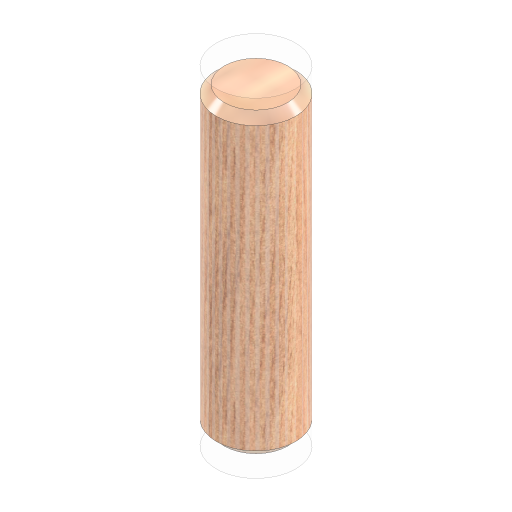
# Autodesk Inventor part: MS Dowel
Saved by Autodesk Inventor 2023 (Build 270158000, 158)
## iProperties
Created: 2024-03-28
Part Number: MS Dowel
Material: Wood (Birch)
Document SubType Name: Modeling
Designer: SauliusD
Density: 0.55 g/cm^3
Appearance: Birch - Natural Polished
Author: SauliusD
Autodesk Inventor part; units mm, degrees
ref_plane "YZ Plane" through (0, 0, 0) normal (1, 0, 0) x (0, 1, 0)
ref_plane "XZ Plane" through (0, 0, 0) normal (0, 1, 0) x (-1, 0, 0)
sketch "Sketch1" plane through (0, 0, 0) normal (0, 0, 1) x (1, 0, 0)
  circle A0 centre (0, 0) radius 4
  dimension "Diam" = 8
  constraints: 1 centre point, 1 coincident
  measures "Diam" diameter of A0
extrude "Extrusion1" add sketch "Sketch1" against normal blind 30
chamfer "Chamfer1" distance 0.8 angle 45 2 edges at (-4, 0, 0) (-4, 0, -30)
ref_plane "Work Plane1" through (0, 0, 1.6) normal (0, 0, 1) x (1, 0, 0)
sketch "Sketch2" plane through (0, 0, 1.6) normal (0, 0, 1) x (1, 0, 0)
  circle A0 centre (0, 0) radius 4 projected
  circle A1 centre (0, 0) radius 4 projected
extrude "Extrusion2" add sketch "Sketch2" against normal blind 33.2 separate body
equation "\"d3\" = 0.1 * Diam"
equation "\"d7\" = L + 2 * Offset"
equation "\"Offset\" = 1.6"
equation "\"d6\" = Offset"
equation "\"L\" = 30"
